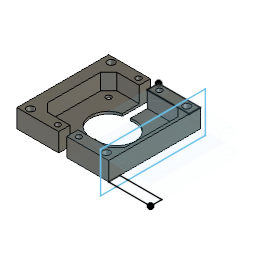
モーター支え(上)(左) (Autodesk Fusion 360 design; units mm, degrees)
Autodesk Fusion 360 part; units mm, degrees
note: some values were not read from the file. Set by a fixed rule: which sketch regions a step uses.
sketch "スケッチ1" plane through (0, 0, 0) normal (0, 0, 1) x (1, 0, 0)
  line L0 (0, 0) -> (52, 0)
  line L1 (52, 0) -> (52, 57)
  line L2 (52, 57) -> (0, 57)
  line L3 (0, 57) -> (0, 0)
  dimension "d1" = 52
  dimension "d2" = 57
  constraint horizontal L0
  constraint vertical L1
  constraint horizontal L2
  constraint vertical L3
  constraint coincident L0.start L3.end
  measures "d1" distance of L0.start L0.end
  measures "d2" distance of L0.start L2.end
extrude "押し出し1" add sketch "スケッチ1" along normal blind 11.5 makes body 1
sketch "スケッチ2" plane through (0, 0, 11.5) normal (0, 0, 1) x (-1, 0, 0)
  line L0 (0, -57) -> (0, 0)
  line L1 (0, 0) -> (-52, 0)
  line L2 (-52, 0) -> (-52, -57)
  line L3 (-52, -57) -> (0, -57)
  line L4 (-45, -7) -> (-45, -50)
  line L5 (-45, -50) -> (-7, -50)
  line L6 (-7, -45) -> (-7, -7)
  line L7 (-12, -7) -> (-45, -7)
  line L8 (-45, -7) -> (-50, -7)
  line L9 (-50, -12) -> (-50, -50)
  line L10 (-50, -50) -> (-45, -50)
  line L11 (-45, -50) -> (-45, -7)
  line L12 (-7, -7) -> (-45, -7)
  line L13 (-50, -7) -> (-50, -45)
  line L14 (-45, -50) -> (-12, -50)
  line L15 (-7, -50) -> (-7, -12)
  line L16 (-7, -45) -> (-12, -50)
  line L17 (-50, -45) -> (-45, -50)
  line L18 (-45, -7) -> (-50, -12)
  line L19 (-7, -12) -> (-12, -7)
  dimension "d6" = 5
  dimension "d7" = 5
  dimension "d8" = 5
  dimension "d9" = 5
  dimension "d10" = 5
  dimension "d11" = 5
  dimension "d12" = 5
  dimension "d13" = 5
  constraint horizontal L8
  constraint vertical L9
  constraint horizontal L10
  constraint vertical L11
  constraint horizontal L12
  constraint vertical L13
  constraint horizontal L14
  constraint vertical L15
  constraint coincident L5.end L14
  constraint coincident L5.end L6
  constraint coincident L9.end L13
  constraint coincident L9.end L14
  constraint coincident L8.end L12
  constraint coincident L8.end L9
  constraint coincident L6.end L15
  constraint coincident L6.end L7
  measures "d6" distance of L5.end L6.start
  measures "d7" distance of L5.end L14.end
  measures "d8" distance of L9.end L13.end
  measures "d9" distance of L9.end L4.end
  measures "d10" distance of L8.end L4.start
  measures "d11" distance of L8.end L9.start
  measures "d12" distance of L6.end L15.end
  measures "d13" distance of L6.end L7.start
extrude "押し出し2" cut sketch "スケッチ2" against normal blind 10 contours L4 L5 L6 L7 L11 L12 L14 L15 L16 L19 | L4 L9 L11 L13 L17 L18 bodies 1
sketch "スケッチ3" plane through (0, 0, 11.5) normal (0, 0, 1) x (-1, 0, 0)
  line L0 (-12, -7) -> (-7, -12)
  line L1 (-7, -12) -> (-7, -45)
  line L2 (-7, -45) -> (-12, -50)
  line L3 (-12, -50) -> (-45, -50)
  line L4 (-45, -50) -> (-50, -45)
  line L5 (-50, -45) -> (-50, -12)
  line L6 (-50, -12) -> (-45, -7)
  line L7 (-45, -7) -> (-12, -7)
  line L8 (0, -57) -> (0, 0)
  line L9 (0, 0) -> (-52, 0)
  line L10 (-52, 0) -> (-52, -57)
  line L11 (-52, -57) -> (0, -57)
  line L12 (0, -57) -> (-52, -57)
  line L13 (-52, -57) -> (-52, -53.5)
  line L14 (-52, -53.5) -> (0, -53.5)
  line L15 (0, -53.5) -> (0, -57)
  line L16 (0, 0) -> (-52, 0)
  line L17 (-52, 0) -> (-52, -3.5)
  line L18 (-52, -3.5) -> (0, -3.5)
  line L19 (0, -3.5) -> (0, 0)
  line L20 (0, 0) -> (-5, 0)
  line L21 (-5, 0) -> (-5, -3.5)
  line L22 (-5, -3.5) -> (0, -3.5)
  line L23 (0, -3.5) -> (0, 0)
  line L24 (-52, 0) -> (-47, 0)
  line L25 (-47, 0) -> (-47, -3.5)
  line L26 (-47, -3.5) -> (-52, -3.5)
  line L27 (-52, -3.5) -> (-52, 0)
  line L28 (0, -57) -> (-5, -57)
  line L29 (-5, -57) -> (-5, -53.5)
  line L30 (-5, -53.5) -> (0, -53.5)
  line L31 (0, -53.5) -> (0, -57)
  line L32 (-52, -57) -> (-47, -57)
  line L33 (-47, -57) -> (-47, -53.5)
  line L34 (-47, -53.5) -> (-52, -53.5)
  line L35 (-52, -53.5) -> (-52, -57)
  line L36 (0, -57) -> (-26, -57)
  line L37 (-26, -57) -> (-26, -53.5)
  line L38 (-26, -53.5) -> (0, -53.5)
  line L39 (0, -53.5) -> (0, -57)
  line L40 (0, 0) -> (-26, 0)
  line L41 (-26, 0) -> (-26, -3.5)
  line L42 (-26, -3.5) -> (0, -3.5)
  line L43 (0, -3.5) -> (0, 0)
  line L44 (-26, 0) -> (-30, 0)
  line L45 (-30, 0) -> (-30, -3.5)
  line L46 (-30, -3.5) -> (-26, -3.5)
  line L47 (-26, -3.5) -> (-26, 0)
  line L48 (-26, 0) -> (-22, 0)
  line L49 (-22, 0) -> (-22, -3.5)
  line L50 (-22, -3.5) -> (-26, -3.5)
  line L51 (-26, -3.5) -> (-26, 0)
  line L52 (-26, -57) -> (-30, -57)
  line L53 (-30, -57) -> (-30, -53.5)
  line L54 (-30, -53.5) -> (-26, -53.5)
  line L55 (-26, -53.5) -> (-26, -57)
  line L56 (-26, -57) -> (-22, -57)
  line L57 (-22, -57) -> (-22, -53.5)
  line L58 (-22, -53.5) -> (-26, -53.5)
  line L59 (-26, -53.5) -> (-26, -57)
  circle A0 centre (-5, -53.5) radius 2.25
  circle A1 centre (-47, -53.5) radius 2.25
  circle A2 centre (-47, -3.5) radius 2.25
  circle A3 centre (-5, -3.5) radius 2.25
  circle A4 centre (-22, -3.5) radius 1.65
  circle A5 centre (-30, -3.5) radius 1.65
  circle A6 centre (-22, -53.5) radius 1.65
  circle A7 centre (-30, -53.5) radius 1.65
  dimension "d16" = 52
  dimension "d17" = 3.5
  dimension "d18" = 52
  dimension "d19" = 3.5
  dimension "d20" = 5
  dimension "d21" = 3.5
  dimension "d22" = 5
  dimension "d23" = 3.5
  dimension "d24" = 5
  dimension "d25" = 3.5
  dimension "d26" = 5
  dimension "d27" = 3.5
  dimension "d28" = 26
  dimension "d29" = 3.5
  dimension "d30" = 26
  dimension "d31" = 3.5
  dimension "d32" = 4
  dimension "d33" = 3.5
  dimension "d34" = 4
  dimension "d35" = 3.5
  dimension "d36" = 4
  dimension "d37" = 4
  dimension "d38" = 3.5
  dimension "d39" = 4.5
  dimension "d40" = 4.5
  dimension "d41" = 4.5
  dimension "d42" = 4.5
  dimension "d43" = 3.3
  dimension "d44" = 3.3
  dimension "d45" = 3.3
  dimension "d46" = 3.3
  constraint horizontal L12
  constraint vertical L13
  constraint horizontal L14
  constraint vertical L15
  constraint coincident L8.start L11.end
  constraint horizontal L16
  constraint vertical L17
  constraint horizontal L18
  constraint vertical L19
  constraint coincident L8.end L9.start
  constraint horizontal L20
  constraint vertical L21
  constraint horizontal L22
  constraint vertical L23
  constraint horizontal L24
  constraint vertical L25
  constraint horizontal L26
  constraint vertical L27
  constraint coincident L9.end L10.start
  constraint horizontal L28
  constraint vertical L29
  constraint horizontal L30
  constraint vertical L31
  constraint horizontal L32
  constraint vertical L33
  constraint horizontal L34
  constraint vertical L35
  constraint horizontal L36
  constraint vertical L37
  constraint horizontal L38
  constraint vertical L39
  constraint horizontal L40
  constraint vertical L41
  constraint horizontal L42
  constraint vertical L43
  constraint horizontal L44
  constraint vertical L45
  constraint horizontal L46
  constraint vertical L47
  constraint horizontal L48
  constraint vertical L49
  constraint horizontal L50
  constraint vertical L51
  constraint horizontal L52
  constraint vertical L53
  constraint horizontal L54
  constraint vertical L55
  constraint horizontal L56
  constraint vertical L57
  constraint horizontal L58
  constraint vertical L59
  constraint coincident L29.end L30.start
  constraint coincident L33.end L34.start
  constraint coincident L25.end L26.start
  constraint coincident L21.end L22.start
  constraint coincident L49.end L50.start
  constraint coincident L45.end L46.start
  constraint coincident L57.end L58.start
  constraint coincident L53.end L54.start
  measures "d16" distance of L8.start L10.end
  measures "d17" distance of L8.start L14.end
  measures "d18" distance of L8.end L9.end
  measures "d19" distance of L8.end L18.end
  measures "d20" distance of L8.end L20.end
  measures "d21" distance of L8.end L18.end
  measures "d22" distance of L9.end L24.end
  measures "d23" distance of L9.end L17.end
  measures "d24" distance of L8.start L28.end
  measures "d25" distance of L8.start L14.end
  measures "d26" distance of L10.end L32.end
  measures "d27" distance of L10.end L13.end
  measures "d28" distance of L8.start L36.end
  measures "d29" distance of L8.start L14.end
  measures "d30" distance of L8.end L40.end
  measures "d31" distance of L8.end L18.end
  measures "d32" distance of L40.end L44.end
  measures "d33" distance of L40.end L41.end
  measures "d34" distance of L40.end L48.end
  measures "d35" distance of L40.end L41.end
  measures "d36" distance of L36.end L52.end
  measures "d37" distance of L36.end L56.end
  measures "d38" distance of L36.end L37.end
  measures "d39" diameter of A0
  measures "d40" diameter of A1
  measures "d41" diameter of A2
  measures "d42" diameter of A3
  measures "d43" diameter of A4
  measures "d44" diameter of A5
  measures "d45" diameter of A6
  measures "d46" diameter of A7
extrude "押し出し3" cut sketch "スケッチ3" against normal blind 11.5 contours L14 L29 L30 L38 A0 | L14 L30 L38 A0 | L14 L29 L38 A0 | L18 L22 L42 A3 | L18 L21 L22 L42 A3 | L14 L38 L57 L58 A6 | L14 L38 L57 A6 | L18 L21 L42 A3 | L14 L38 L58 A6 | L18 L42 L50 A4 | L18 L42 L49 A4 | L14 L53 A7 | L14 L53 L54 A7 | L14 L54 A7 | L18 L42 L49 L50 A4 | L14 L33 L34 A1 | L14 L33 A1 | L14 L34 A1 | L18 L45 L46 A5 | L18 L45 A5 | L18 L46 A5 | L18 L25 A2 | L18 L25 L26 A2 | L18 L26 A2 bodies 1
sketch "スケッチ4" plane through (0, 0, 11.5) normal (0, 0, 1) x (-1, 0, 0)
  circle A0 centre (-30, -3.5) radius 1.65
  circle A1 centre (-22, -53.5) radius 1.65
  circle A2 centre (-30, -53.5) radius 1.65
  circle A3 centre (-22, -3.5) radius 1.65
  circle A4 centre (-47, -3.5) radius 2.25
  circle A5 centre (-5, -53.5) radius 2.25
  circle A6 centre (-47, -53.5) radius 2.25
  circle A7 centre (-5, -3.5) radius 2.25
  line L0 (-12, -7) -> (-7, -12)
  line L1 (-7, -12) -> (-7, -45)
  line L2 (-7, -45) -> (-12, -50)
  line L3 (-12, -50) -> (-45, -50)
  line L4 (-45, -50) -> (-50, -45)
  line L5 (-50, -45) -> (-50, -12)
  line L6 (-50, -12) -> (-45, -7)
  line L7 (-45, -7) -> (-12, -7)
  line L8 (0, -57) -> (0, 0)
  line L9 (0, 0) -> (-52, 0)
  line L10 (-52, 0) -> (-52, -57)
  line L11 (-52, -57) -> (0, -57)
  line L12 (0, -57) -> (-26, -57)
  line L13 (-26, -57) -> (-26, -50)
  line L14 (-26, -50) -> (0, -50)
  line L15 (0, -50) -> (0, -57)
  dimension "d49" = 26
  dimension "d50" = 7
  constraint horizontal L12
  constraint vertical L13
  constraint horizontal L14
  constraint vertical L15
  constraint coincident L8.start L11.end
  measures "d49" distance of L8.start L12.end
  measures "d50" distance of L8.start L14.end
sketch "スケッチ5" plane through (0, 0, 0) normal (0, 0, -1) x (1, 0, 0)
  circle A0 centre (30, -3.5) radius 1.65
  circle A1 centre (22, -53.5) radius 1.65
  circle A2 centre (30, -53.5) radius 1.65
  circle A3 centre (22, -3.5) radius 1.65
  circle A4 centre (47, -3.5) radius 2.25
  circle A5 centre (5, -53.5) radius 2.25
  circle A6 centre (47, -53.5) radius 2.25
  circle A7 centre (5, -3.5) radius 2.25
  line L0 (0, 0) -> (0, -57)
  line L1 (0, -57) -> (52, -57)
  line L2 (52, -57) -> (52, 0)
  line L3 (52, 0) -> (0, 0)
  line L4 (52, 0) -> (26, 0)
  line L5 (26, 0) -> (26, -7)
  line L6 (26, -7) -> (52, -7)
  line L7 (52, -7) -> (52, 0)
  dimension "d51" = 26
  dimension "d52" = 7
  constraint horizontal L4
  constraint vertical L5
  constraint horizontal L6
  constraint vertical L7
  constraint coincident L2.end L3.start
  measures "d51" distance of L2.end L4.end
  measures "d52" distance of L2.end L6.end
ref_plane "作業平面1" through (26, 0, 0) normal (1, 0, 0) x (0, 1, 0)
sketch "スケッチ6" plane through (26, 0, 0) normal (1, 0, 0) x (0, 1, 0)
  line L0 (-5, -5) -> (60, -5)
  line L1 (60, -5) -> (60, 20)
  line L2 (60, 20) -> (-5, 20)
  line L3 (-5, 20) -> (-5, -5)
  constraint horizontal L0
  constraint vertical L1
  constraint horizontal L2
  constraint vertical L3
sketch "スケッチ7" plane through (26, 0, 0) normal (1, 0, 0) x (0, 1, 0)
sketch "スケッチ8" plane through (0, 0, 11.5) normal (0, 0, 1) x (-1, 0, 0)
  line L0 (-50, -30) -> (-28.5, -30)
  line L1 (-27, -7) -> (-27, -28.5)
  circle A0 centre (-28.5, -28.5) radius 11.25
  line L2 (-50, -7) -> (-44, -7)
  line L3 (-44, -7) -> (-44, -13)
  line L4 (-44, -13) -> (-50, -13)
  line L5 (-50, -13) -> (-50, -7)
  line L6 (-7, -7) -> (-13, -7)
  line L7 (-13, -7) -> (-13, -13)
  line L8 (-13, -13) -> (-7, -13)
  line L9 (-7, -13) -> (-7, -7)
  line L10 (-50, -50) -> (-44, -50)
  line L11 (-44, -50) -> (-44, -44)
  line L12 (-44, -44) -> (-50, -44)
  line L13 (-50, -44) -> (-50, -50)
  line L14 (-7, -50) -> (-13, -50)
  line L15 (-13, -50) -> (-13, -44)
  line L16 (-13, -44) -> (-7, -44)
  line L17 (-7, -44) -> (-7, -50)
  circle A1 centre (-44, -13) radius 1.65
  circle A2 centre (-13, -13) radius 1.65
  circle A3 centre (-44, -44) radius 1.65
  circle A4 centre (-13, -44) radius 1.65
  dimension "d53" = 22.5
  dimension "d58" = 3.3
  dimension "d59" = 3.3
  dimension "d60" = 3.3
  dimension "d61" = 3.3
  constraint horizontal L0
  constraint perpendicular L0 L1
  constraint horizontal L2
  constraint vertical L3
  constraint horizontal L4
  constraint vertical L5
  constraint horizontal L6
  constraint vertical L7
  constraint horizontal L8
  constraint vertical L9
  constraint horizontal L10
  constraint vertical L11
  constraint horizontal L12
  constraint vertical L13
  constraint horizontal L14
  constraint vertical L15
  constraint horizontal L16
  constraint vertical L17
  constraint coincident L3.end L4.start
  constraint coincident L7.end L8.start
  constraint coincident L11.end L12.start
  constraint coincident L15.end L16.start
  measures "d53" diameter of A0
  measures "d58" diameter of A1
  measures "d59" diameter of A2
  measures "d60" diameter of A3
  measures "d61" diameter of A4
extrude "押し出し4" cut sketch "スケッチ8" against normal blind 11.5 contours A0 | L3 L4 A1 | L3 L4 A1 | L7 L8 A2 | L7 L8 A2 | L11 L12 A3 | L11 L12 A3 | L15 L16 A4 | L15 L16 A4 bodies 1
move_body "移動1" bodies 1 to x (1, 0, 0) y (0, 1, 0) z (0, 0, 1) at (-26, 0, 0)
split "分割1" by plane through (0, 0, 0) normal (1, 0, 0) bodies 1 makes body 2 at (9.3365, 45.1425, 0)
move_body "移動2" bodies 1 to x (1, 0, 0) y (0, 1, 0) z (0, 0, 1) at (-5, 0, 0)
equation "d7 = d6"
equation "d9 = d8"
equation "d11 = d10"
equation "d13 = d12"
